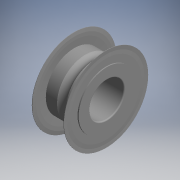
# Autodesk Inventor part: SKF_W 619/3-2Z_PART1
Saved by Autodesk Inventor 2021.3 (Build 253353000, 353)
## iProperties
Part Number: SKF_W 619/3-2Z_PART1
Material: Generic
Catalog Web Link: www.cadenas.de
Description: -Deep groove ball bearings
Vendor: SKF
Document SubType Name: Modeling
Designer: partserver
Manufacturer: SKF
Mass: 1 g
Surface Area: 1.944 cm^2
Volume: 0.0385157 cm^3
Density: 1 g/cm^3
Appearance: PSOLRGB-175-175-175
Category: PARTsolutions
Company: SKF
PSOL_IDENT_0: {$CADENAS_DATA\23d-libs\skf\bearings_units_and_housings\ball_bearings\deep_groove_ball_bearings\bb1_
PSOL_IDENT_1: 001_101.prj},207 {VTYP=3D},{NB=SKF_W 619/3-2Z_PART1},{LINA=SKF_W 619/3-2Z_PART1},{NN=BB1_001_101_PAR
PSOL_IDENT_2: T1},{NOPRJ=TRUE},{DATE=13.05.2022 09:20:28},{GEOMDATE=02.05.2022 07:22:49},{VERSION=},{LINEID=17690}
PSOL_IDENT_3: ,{WBVAR=},{WBNUMERIC=}  {NB=SKF_W 619/3-2Z_PART1},{LINA=SKF_W 619/3-2Z_PART1},{KT=DUMMY},{DESIGNATIO
PSOL_IDENT_4: N=W 619/3-2Z},{R12=0.10},{DD=3.000},{D=8.000},{B=3.000},{C=},{CX=},{CXX=},{CA=0.000},{XXVARIANT=},{X
PSOL_IDENT_5: XDESIGN=Single row stainless steel},{XXSEALING=Shield on both sides},{DESIGN=dgbbw2z},{DESIGNIR=dgbb
PSOL_IDENT_6: w2z},{VARIANT=},{DD1=5.00},{DD2=5},{DD2X=},{DD2A=5.00},{D1=6.80},{D1X=0.00},{D2=7.4},{D2A=7.40},{D3=
PSOL_IDENT_7: },{D3X=},{D3A=0.000},{D4=},{HH=0.000},{BB=0.000},{BBX=},{BBA=0.000},{FF=},{R0MAX=0.000},{R0=0.000},{
PSOL_IDENT_8: PITCH=5.90},{DW=1.200},{DDAMIN=3.800},{DDAMAX=4.900},{DDBMIN=0.000},{DDBMAX=0.000},{DBMIN=0.000},{DA
PSOL_IDENT_9: MAX=7.500},{BBAMIN=0.000},{CAMAX=0.000},{RAMAX=0.100},{LOAD1=0.225},{LOAD2=0.072},{LOAD3=0.003},{SPE
PSOL_IDENT_10: ED1=150000},{SPEED2=75000},{KR=0.025},{F0=7.200},{Z=7},{II=1},{MASS=0.001},{BEARING=W 619/3-2Z},{RIN
PSOL_IDENT_11: G=},{HELP=0.600},{HELP2=0.300},{DD1ALG=2.500},{YALG=2.500},{PITCH1=5.900},{DW1=1.200},{YALG1=3.400},
PSOL_IDENT_12: {HALG1=0.600},{SH=2.500},{CU=0.360},{HALG=1},{B1=0},{SHIELDHELP=2},{D4A=0.000},{FFA=0.000},{RS1=},{H
PSOL_IDENT_13: ELP3=0}
NB: SKF_W 619/3-2Z_PART1
NT: Deep groove ball bearings
NBSYN: SKF_$DESIGNATION._PART1
LINA: SKF_W 619/3-2Z_PART1
CATALOG: SKF
DESIGNATION: W 619/3-2Z
R12: 0.1
DD: 3
D: 8
B: 3
XXDESIGN: Single row stainless steel
XXSEALING: Shield on both sides
DD2: 5
D2: 7.4
LOAD1: 0.225
LOAD2: 0.072
LOAD3: 0.003
SPEED1: 150000
SPEED2: 75000
BEARING: W 619/3-2Z
SUPPLIER: SKF
ARTICLENO: SKF_W 619/3-2Z_PART1
BOMINFO: SKF_W 619/3-2Z_PART1
CREATOR: CADENAS GmbH
Title: SKF_W 619/3-2Z_PART1
Author: Cadenas PARTsolutions
Comments: Deep groove ball bearings
Autodesk Inventor part; units mm, degrees
ref_plane "YZ Plane" through (0, 0, 0) normal (1, 0, 0) x (0, 1, 0)
ref_plane "XZ Plane" through (0, 0, 0) normal (0, 1, 0) x (-1, 0, 0)
ref_plane "XY Plane" through (0, 0, 0) normal (0, 0, 1) x (1, 0, 0)
sketch "Sketch_18" plane through (0, 0, 0) normal (0, 0, 1) x (1, 0, 0)
  line L0 (50, 0) -> (-50, 0)
  arc A0 (0, 1.6) -> (0.1, 1.5) centre (0.1, 1.6) ccw
  line L1 (0.1, 1.5) -> (2.9, 1.5)
  arc A1 (2.9, 1.5) -> (3, 1.6) centre (2.9, 1.6) ccw
  line L2 (3, 1.6) -> (3, 2.5)
  line L3 (3, 2.5) -> (1.8969, 2.5)
  arc A2 (1.1031, 2.5) -> (1.8969, 2.5) centre (1.5, 2.95) ccw
  line L4 (1.1031, 2.5) -> (0, 2.5)
  line L5 (0, 2.5) -> (0, 1.6)
  constraints: 12 end point, 6 point on circle, 3 centre point
revolve "Revolution1" add sketch "Sketch_18" angle 360 about axis through (50, 0, 0) along (1, 0, 0)
sketch "Sketch_20" plane through (0, 0, 0) normal (0, 0, 1) x (1, 0, 0)
  line L0 (50, 0) -> (-50, 0)
  line L1 (0.09, 3.7) -> (0.105, 3.3975)
  line L2 (0.105, 3.3975) -> (0.09, 3.095)
  line L3 (0.09, 3.095) -> (0.09, 2.49)
  line L4 (0.09, 2.49) -> (0.12, 2.49)
  line L5 (0.12, 2.49) -> (0.15, 3.095)
  line L6 (0.15, 3.095) -> (0.15, 3.3975)
  line L7 (0.15, 3.3975) -> (0.12, 3.7)
  line L8 (0.12, 3.7) -> (0.09, 3.7)
  constraints: 18 end point
revolve "Revolution2" add sketch "Sketch_20" angle 360 about axis through (50, 0, 0) along (1, 0, 0)
sketch "Sketch_21" plane through (0, 0, 0) normal (0, 0, 1) x (1, 0, 0)
  line L0 (50, 0) -> (-50, 0)
  line L1 (2.85, 3.3975) -> (2.85, 3.095)
  line L2 (2.85, 3.095) -> (2.88, 2.49)
  line L3 (2.88, 2.49) -> (2.91, 2.49)
  line L4 (2.91, 2.49) -> (2.91, 3.095)
  line L5 (2.91, 3.095) -> (2.895, 3.3975)
  line L6 (2.895, 3.3975) -> (2.91, 3.7)
  line L7 (2.91, 3.7) -> (2.88, 3.7)
  line L8 (2.88, 3.7) -> (2.85, 3.3975)
  constraints: 18 end point
revolve "Revolution3" add sketch "Sketch_21" angle 360 about axis through (50, 0, 0) along (1, 0, 0)
body "Solid1"
